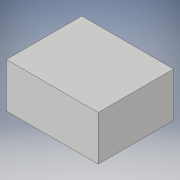
# Autodesk Inventor part: shaft toothed clip holder v2 hole bool
Saved by Autodesk Inventor 2019.3 (Build 233278000, 278)
## iProperties
Created: 2018-12-21
Part Number: shaft toothed clip holder v2 hole bool
Material: Generic
Document SubType Name: Modeling
Designer: Frienddo
Density: 1 g/cm^3
Appearance: Default
Author: Frienddo
Autodesk Inventor part; units mm, degrees
ref_plane "YZ Plane" through (0, 0, 0) normal (1, 0, 0) x (0, 1, 0)
ref_plane "XZ Plane" through (0, 0, 0) normal (0, 1, 0) x (-1, 0, 0)
ref_plane "XY Plane" through (0, 0, 0) normal (0, 0, 1) x (1, 0, 0)
sketch "Sketch1" plane through (0, 0, 0) normal (0, 1, 0) x (-1, 0, 0)
  line L0 (-14.927, -12.25) -> (14.927, -12.25)
  line L1 (14.927, -12.25) -> (14.927, 12.25)
  line L2 (14.927, 12.25) -> (-14.927, 12.25)
  line L3 (-14.927, 12.25) -> (-14.927, -12.25)
  line L4 (-14.927, -12.25) -> (14.927, 12.25) construction
  line L5 (14.927, -12.25) -> (-14.927, 12.25) construction
  point P0 (0, 0)
  dimension "d0" = 29.854
  dimension "d1" = 24.5
  constraints: 12 end point, 2 midpoint, 2 parallel, 1 horizontal, 1 perpendicular
  measures "d0" distance of L1.end L2.end
  measures "d1" distance of L0.end L1.end
extrude "Extrusion1" add sketch "Sketch1" along normal mid plane 14.5
body "Solid1"
